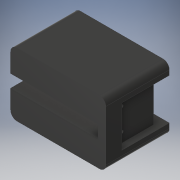
# Autodesk Inventor part: GA01
Saved by Autodesk Inventor 2017 (Build 210142000, 142)
## iProperties
Created: 2018-10-23
Part Number: GA01
Material: ABS Plastic
Document SubType Name: Modeling
Designer: Dell
Density: 1.06 g/cm^3
Appearance: Smooth - Black
Author: Dell
Autodesk Inventor part; units mm, degrees
ref_plane "YZ Plane" through (0, 0, 0) normal (1, 0, 0) x (0, 1, 0)
ref_plane "XZ Plane" through (0, 0, 0) normal (0, 1, 0) x (-1, 0, 0)
ref_plane "XY Plane" through (0, 0, 0) normal (0, 0, 1) x (1, 0, 0)
sketch "Sketch1" plane through (0, 0, 0) normal (0, 0, 1) x (1, 0, 0)
  line L0 (0, 0) -> (150, 0)
  line L1 (150, 0) -> (150, 100)
  line L2 (150, 100) -> (0, 100)
  line L3 (0, 100) -> (0, 0)
  dimension "d0" = 150
  dimension "d1" = 100
  constraints: 8 end point, 2 parallel, 1 horizontal, 1 perpendicular
  measures "d0" distance of L2.end L1.end
  measures "d1" distance of L1.end L0.end
extrude "Extrusion1" add sketch "Sketch1" along normal blind 100
fillet "Fillet1" radius 10 4 edges at (150, 100, 50) (150, 0, 50) (0, 100, 50) (0, 0, 50)
sketch "Sketch2" plane through (0, 0, 0) normal (0, 0, -1) x (-1, 0, 0)
  circle A0 centre (-75, 50) radius 2.5
  circle A1 centre (-45, 50) radius 2.5
  line L0 (-140, 100) -> (-10, 100) projected
  line L1 (0, 90) -> (0, 10) projected
  circle A2 centre (-60, 75.9808) radius 2.5
  circle A3 centre (-90, 75.9808) radius 2.5
  circle A4 centre (-105, 50) radius 2.5
  circle A5 centre (-90, 24.0192) radius 2.5
  circle A6 centre (-60, 24.0192) radius 2.5
  point P0 (0, 0)
  point P1 (-75, 100)
  point P2 (0, 50)
  dimension "d5" = 5
  dimension "d6" = 5
  dimension "d7" = 30
  dimension "d10" = 360
  constraints: 7 centre point, 2 horizontal alignment, 2 midpoint, 1 vertical alignment, 13 other
  measures "d5" diameter of A0
  measures "d6" diameter of A1
  measures "d7" distance of A1.centre A0.centre
extrude "Extrusion2" cut sketch "Sketch2" against normal blind 25
sketch "Sketch3" plane through (0, 0, 100) normal (0, 0, 1) x (1, 0, 0)
  line L0 (12.5, 40) -> (137.5, 40)
  line L1 (137.5, 40) -> (137.5, 60)
  line L2 (137.5, 60) -> (12.5, 60)
  line L3 (12.5, 60) -> (12.5, 40)
  line L4 (10, 0) -> (140, 0) projected
  line L5 (0, 90) -> (0, 10) projected
  point P0 (0, 0)
  point P1 (75, 40)
  point P2 (75, 0)
  point P3 (12.5, 50)
  point P4 (0, 50)
  dimension "d14" = 20
  dimension "d15" = 125
  constraints: 8 end point, 4 midpoint, 2 parallel, 1 horizontal, 1 horizontal alignment, 1 perpendicular, 1 vertical alignment
  measures "d14" distance of L2.end L0.start
  measures "d15" distance of L0.start L0.end
extrude "Extrusion3" cut sketch "Sketch3" against normal blind 50
sketch "Sketch4" plane through (0, 0, 50) normal (0, 0, 1) x (1, 0, 0)
  line L0 (100, 34.5) -> (50, 34.5)
  line L1 (50, 34.5) -> (50, 65.5)
  line L2 (50, 65.5) -> (100, 65.5)
  line L3 (100, 65.5) -> (100, 34.5)
  line L4 (150, 10) -> (150, 90) projected
  line L5 (10, 0) -> (140, 0) projected
  point P0 (0, 0)
  point P1 (100, 50)
  point P2 (150, 50)
  point P3 (75, 34.5)
  point P4 (75, 0)
  dimension "d18" = 50
  dimension "d19" = 31
  constraints: 8 end point, 4 midpoint, 2 parallel, 1 horizontal, 1 horizontal alignment, 1 perpendicular, 1 vertical alignment
  measures "d18" distance of L1.end L2.end
  measures "d19" distance of L0.end L1.end
extrude "Extrusion4" cut sketch "Sketch4" against normal through all
sketch "Sketch5" plane through (0, 0, 100) normal (0, 0, 1) x (1, 0, 0)
  line L0 (68, 63.5) -> (92, 63.5) construction
  line L1 (92, 63.5) -> (92, 36.5) construction
  line L2 (92, 36.5) -> (68, 36.5) construction
  line L3 (68, 36.5) -> (68, 63.5) construction
  line L4 (0, 90) -> (0, 10) projected
  line L5 (140, 100) -> (10, 100) projected
  circle A0 centre (68, 63.5) radius 1.5
  circle A1 centre (68, 36.5) radius 1.5
  circle A2 centre (92, 36.5) radius 1.5
  circle A3 centre (92, 63.5) radius 1.5
  circle A4 centre (76, 63.5) radius 1.5
  circle A5 centre (84, 63.5) radius 1.5
  circle A6 centre (76, 36.5) radius 1.5
  circle A7 centre (84, 36.5) radius 1.5
  line L6 (50, 40) -> (50, 60) projected
  line L7 (100, 60) -> (100, 40) projected
  point P0 (0, 0)
  point P1 (68, 50)
  point P2 (0, 50)
  point P3 (80, 63.5)
  point P4 (75, 100)
  dimension "d22" = 24
  dimension "d23" = 27
  dimension "d24" = 3
  dimension "d25" = 3
  dimension "d26" = 3
  dimension "d27" = 3
  dimension "d28" = 3
  dimension "d29" = 3
  dimension "d30" = 3
  dimension "d31" = 3
  dimension "d32" = 8
  dimension "d33" = 8
  dimension "d37" = 8
  constraints: 8 centre point, 8 end point, 4 coincident, 4 midpoint, 4 point on line, 2 parallel, 2 vertical alignment, 1 horizontal, 1 horizontal alignment, 1 perpendicular
  measures "d22" distance of L1.end L2.end
  measures "d23" distance of L0.end L1.end
  measures "d24" diameter of A0
  measures "d25" diameter of A1
  measures "d26" diameter of A2
  measures "d27" diameter of A3
  measures "d28" diameter of A4
  measures "d29" diameter of A5
  measures "d30" diameter of A6
  measures "d31" diameter of A7
  measures "d32" distance of L1.end A7.centre
  measures "d33" distance of L2.end A6.centre
  measures "d37" distance between parallel lines of L7 L1
extrude "Extrusion5" cut sketch "Sketch5" against normal through all
sketch "Sketch7" plane through (0, 0, 0) normal (0, 0, -1) x (-1, 0, 0)
  line L0 (-100, 34.5) -> (-100, 65.5) projected
  line L1 (-100, 65.5) -> (-50, 65.5) projected
  line L2 (-150, 10) -> (-150, 90) projected
  line L3 (0, 90) -> (0, 10) projected
  line L4 (-150, 82.5) -> (0, 82.5)
  line L5 (0, 82.5) -> (0, 17.5)
  line L6 (0, 17.5) -> (-150, 17.5)
  line L7 (-150, 17.5) -> (-150, 82.5)
  point P0 (0, 0)
  point P1 (-75, 50)
  point P2 (-100, 50)
  point P3 (-75, 65.5)
  point P4 (-150, 50)
  point P5 (-150, 50)
  point P6 (-150, 50)
  dimension "d55" = 65
  constraints: 8 end point, 5 midpoint, 2 horizontal alignment, 2 parallel, 2 point on line, 1 coincident, 1 horizontal, 1 perpendicular, 1 vertical alignment
  measures "d55" distance between parallel lines of L6 L4
extrude "Extrusion6" cut sketch "Sketch7" against normal blind 15
sketch "Sketch8" plane through (0, 0, 15) normal (0, 0, -1) x (-1, 0, 0)
  line L0 (-110, 75) -> (-130, 75)
  line L1 (-130, 75) -> (-130, 25)
  line L2 (-130, 25) -> (-110, 25)
  line L3 (-110, 25) -> (-110, 75)
  line L4 (-100, 65.5) -> (-100, 34.5) projected
  point P0 (0, 0)
  point P1 (-110, 50)
  point P2 (-100, 50)
  dimension "d56" = 10
  dimension "d57" = 20
  dimension "d60" = 50
  constraints: 8 end point, 2 midpoint, 2 parallel, 1 horizontal, 1 horizontal alignment, 1 perpendicular
  measures "d56" distance between parallel lines of L3 L4
  measures "d57" distance of L0.start L0.end
  measures "d60" distance of L0.end L1.end
extrude "Extrusion7" cut sketch "Sketch8" against normal blind 20
sketch "Sketch9" plane through (0, 0, 15) normal (0, 0, -1) x (-1, 0, 0)
  line L0 (-110, 75) -> (-110, 25) projected
  line L1 (-100, 65.5) -> (-100, 34.5) projected
  line L2 (-110, 60) -> (-100, 60)
  line L3 (-100, 60) -> (-100, 55)
  line L4 (-100, 55) -> (-110, 55)
  line L5 (-110, 55) -> (-110, 60)
  circle A0 centre (-105, 50) radius 2.5 construction
  line L6 (-110, 45) -> (-100, 45)
  line L7 (-100, 45) -> (-100, 40)
  line L8 (-100, 40) -> (-110, 40)
  line L9 (-110, 40) -> (-110, 45)
  point P0 (0, 0)
  dimension "d61" = 5
  dimension "d62" = 5
  dimension "d63" = 5
  dimension "d64" = 5
  constraints: 16 end point, 4 parallel, 4 point on line, 2 horizontal, 2 perpendicular
  measures "d61" distance from line of L4 A0.centre
  measures "d62" distance between parallel lines of L4 L2
  measures "d63" distance between parallel lines of L8 L6
  measures "d64" distance from line of A0.centre L6
extrude "Extrusion8" cut sketch "Sketch9" against normal blind 5 contours L2 L1 L4 L0 | L6 L1 L8 L0
sketch "Sketch10" plane through (0, 0, 15) normal (0, 0, -1) x (-1, 0, 0)
  line L0 (-50, 34.5) -> (-50, 65.5) projected
  circle A0 centre (-45, 50) radius 2.5 projected
  line L1 (-40, 75) -> (-20, 75)
  line L2 (-20, 75) -> (-20, 25)
  line L3 (-20, 25) -> (-40, 25)
  line L4 (-40, 25) -> (-40, 75)
  point P0 (0, 0)
  point P1 (-40, 50)
  dimension "d67" = 20
  dimension "d68" = 50
  dimension "d69" = 10
  constraints: 8 end point, 2 parallel, 1 horizontal, 1 horizontal alignment, 1 midpoint, 1 perpendicular
  measures "d67" distance of L1.start L1.end
  measures "d68" distance of L1.end L2.end
  measures "d69" distance between parallel lines of L4 L0
extrude "Extrusion9" cut sketch "Sketch10" against normal blind 20 contours L1 L2 L3 L4
sketch "Sketch11" plane through (0, 0, 15) normal (0, 0, -1) x (-1, 0, 0)
  line L0 (-50, 34.5) -> (-50, 65.5) projected
  line L1 (-50, 55) -> (-40, 55)
  line L2 (-40, 55) -> (-40, 60)
  line L3 (-40, 60) -> (-50, 60)
  line L4 (-50, 60) -> (-50, 55)
  line L5 (-50, 45) -> (-40, 45)
  line L6 (-40, 45) -> (-40, 40)
  line L7 (-40, 40) -> (-50, 40)
  line L8 (-50, 40) -> (-50, 45)
  line L9 (-40, 25) -> (-40, 75) projected
  point P0 (0, 0)
  point P1 (-100, 45)
  point P2 (-100, 40)
  point P3 (-100, 55)
  point P4 (-100, 60)
  constraints: 16 end point, 4 horizontal alignment, 4 parallel, 4 point on line, 2 horizontal, 2 perpendicular
extrude "Extrusion10" cut sketch "Sketch11" against normal blind 5 contours L0 L5 L6 L7 | L0 L3 L2 L1
sketch "Sketch12" plane through (0, 0, 100) normal (0, 0, 1) x (1, 0, 0)
  circle A0 centre (92, 36.5) radius 1.5 projected
  circle A1 centre (84, 36.5) radius 1.5 projected
  circle A2 centre (76, 36.5) radius 1.5 projected
  circle A3 centre (68, 36.5) radius 1.5 projected
  circle A4 centre (68, 63.5) radius 1.5 projected
  circle A5 centre (76, 63.5) radius 1.5 projected
  circle A6 centre (84, 63.5) radius 1.5 projected
  circle A7 centre (92, 63.5) radius 1.5 projected
  point P0 (0, 0)
extrude "Extrusion11" add sketch "Sketch12" against normal blind 10
sketch "Sketch13" plane through (0, 0, 15) normal (0, 0, -1) x (-1, 0, 0)
  line L0 (-150, 17.5) -> (-150, 82.5) projected
  line L1 (0, 82.5) -> (0, 17.5) projected
  line L2 (0, 17.5) -> (-150, 17.5) projected
  line L3 (-150, 82.5) -> (-140, 82.5)
  line L4 (-140, 82.5) -> (-140, 17.5)
  line L5 (-140, 17.5) -> (-150, 17.5)
  line L6 (-150, 17.5) -> (-150, 82.5)
  line L7 (0, 82.5) -> (-10, 82.5)
  line L8 (-10, 82.5) -> (-10, 17.5)
  line L9 (-10, 17.5) -> (0, 17.5)
  line L10 (0, 17.5) -> (0, 82.5)
  point P0 (0, 0)
  dimension "d76" = 10
  dimension "d77" = 10
  constraints: 16 end point, 4 parallel, 2 horizontal, 2 perpendicular, 2 point on line
  measures "d76" distance between parallel lines of L0 L4
  measures "d77" distance between parallel lines of L1 L8
extrude "Extrusion12" cut sketch "Sketch13" against normal blind 60
sketch "Sketch14" plane through (140, 17.5, 15) normal (1, 0, 0) x (0, 0, -1)
  circle A0 centre (-50, 15) radius 2.5
  circle A1 centre (-50, 50) radius 2.5
  line L0 (-50, 15) -> (-50, 50) construction
  line L1 (-60, 0) -> (-60, 65) projected
  point P0 (15, -17.5)
  point P1 (-50, 32.5)
  point P2 (-60, 32.5)
  dimension "d80" = 5
  dimension "d81" = 5
  dimension "d82" = 10
  dimension "d83" = 35
  constraints: 2 centre point, 2 end point, 2 midpoint, 1 horizontal alignment, 1 vertical
  measures "d80" diameter of A0
  measures "d81" diameter of A1
  measures "d82" distance between parallel lines of L1 L0
  measures "d83" distance of L0.start L0.end
extrude "Extrusion13" cut sketch "Sketch14" against normal blind 25
sketch "Sketch15" plane through (10, 17.5, 15) normal (-1, 0, 0) x (0, 0, 1)
  circle A0 centre (50, 50) radius 2.5 projected
  circle A1 centre (50, 15) radius 2.5 projected
  point P0 (-15, -17.5)
extrude "Extrusion14" cut sketch "Sketch15" against normal blind 25
sketch "Sketch16" plane through (137.5, 40, 100) normal (-1, 0, 0) x (0, 0, 1)
  line L0 (0, 20) -> (0, 0) projected
  line L1 (0, 20) -> (-50, 20) projected
  line L2 (-50, 20) -> (-50, 0) projected
  line L3 (0, 0) -> (-50, 0) projected
  circle A0 centre (-45, -17) radius 6.5
  line L4 (0, -40) -> (-100, -40) projected
  circle A1 centre (-45, 37) radius 6.5
  line L5 (-100, 60) -> (0, 60) projected
  line L6 (-39.5, 37) -> (-50.5, 37)
  line L7 (-50.5, 37) -> (-50.5, -17)
  line L8 (-50.5, -17) -> (-39.5, -17)
  line L9 (-39.5, -17) -> (-39.5, 37)
  line L10 (-100, 42.5) -> (-25, 42.5) projected
  line L11 (-25, -22.5) -> (-100, -22.5) projected
  line L12 (-39.5, -17) -> (-50.5, -17)
  line L13 (-50.5, -17) -> (-50.5, 0)
  line L14 (-50.5, 0) -> (-39.5, 0)
  line L15 (-39.5, 0) -> (-39.5, -17)
  line L16 (-50.5, 37) -> (-39.5, 37)
  line L17 (-39.5, 37) -> (-39.5, 20)
  line L18 (-39.5, 20) -> (-50.5, 20)
  line L19 (-50.5, 20) -> (-50.5, 37)
  dimension "d88" = 13
  dimension "d90" = 5
  dimension "d91" = 13
  dimension "d92" = 5
  dimension "d94" = 11
  dimension "d97" = 5.5
  dimension "d98" = 5.5
  constraints: 24 end point, 6 parallel, 3 horizontal, 3 perpendicular, 3 point on line, 2 centre point, 2 midpoint, 1 coincident, 1 horizontal alignment
  measures "d88" diameter of A0
  measures "d90" distance from line of L2 A0.centre
  measures "d91" diameter of A1
  measures "d92" distance from line of L2 A1.centre
  measures "d94" distance of L8.end L7.end
  measures "d97" distance from line of L11 A0.centre
  measures "d98" distance between parallel lines of L10 L6
extrude "Extrusion15" cut sketch "Sketch16" along normal through all contours L1 L18 L7 A1 L9 | L9 A0 L7 L14 L3 | L9 L6 L7 A1 L10 | A1 L7 L6 L9 | L9 L8 L7 A0 | A0 L11 L7 L8 L9 | A1 L10 | A0 L11
sketch "Sketch19" plane through (137.5, 40, 100) normal (-1, 0, 0) x (0, 0, 1)
  line L0 (0, 20) -> (0, 0) projected
  line L1 (0, 20) -> (-39.5, 20) projected
  line L2 (-39.5, 20) -> (-39.5, 33.5359) projected
  arc A0 (-39.5, 33.5359) -> (-50.5, 33.5359) centre (-45, 37) ccw projected
  line L3 (-50.5, 33.5359) -> (-50.5, 20) projected
  line L4 (-50.5, 20) -> (-50, 20) projected
  line L5 (-50, 20) -> (-50, 0) projected
  line L6 (-50, 0) -> (-50.5, 0) projected
  line L7 (-50.5, 0) -> (-50.5, -13.5359) projected
  arc A1 (-50.5, -13.5359) -> (-39.5, -13.5359) centre (-45, -17) ccw projected
  line L8 (-39.5, -13.5359) -> (-39.5, 0) projected
  line L9 (0, 0) -> (-39.5, 0) projected
  point P0 (-100, -40)
extrude "Extrusion16" cut sketch "Sketch19" along normal through all
body "Solid1"
